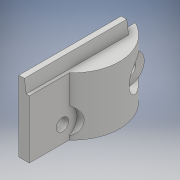
# Autodesk Inventor part: Faceplatev11
Saved by Autodesk Inventor 2017 (Build 210142000, 142)
## iProperties
Created: 2017-12-13
Part Number: Faceplatev11
Material: Generic
Document SubType Name: Modeling
Designer: andrew
Density: 1 g/cm^3
Appearance: Default
Author: andrew
Autodesk Inventor part; units mm, degrees
ref_plane "YZ Plane" through (0, 0, 0) normal (1, 0, 0) x (0, 1, 0)
ref_plane "XZ Plane" through (0, 0, 0) normal (0, 1, 0) x (-1, 0, 0)
ref_plane "XY Plane" through (0, 0, 0) normal (0, 0, 1) x (1, 0, 0)
sketch "Sketch1" plane through (0, 0, 0) normal (0, 0, 1) x (1, 0, 0)
  arc A0 (2, -4.031129) -> (2, 4.031129) centre (0, 0) ccw
  line L0 (2, -4.031129) -> (2, -1.999397)
  line L1 (2, 2.000654) -> (2, 4.031129)
  line L2 (2, 2.000654) -> (2, -1.999397)
  constraints: 6 end point, 2 point on circle, 1 centre point, 1 vertical
extrude "Extrusion1" add sketch "Sketch1" along normal blind 7.3
sketch "Sketch2" plane through (0, 0, 7.3) normal (0, 0, 1) x (1, 0, 0)
  arc A0 (2, -4.031129) -> (2, 4.031129) centre (0, 0) ccw
  line L0 (2, 4.031129) -> (2, 2.681129)
  line L1 (2, 4.031129) -> (2, -4.031129)
  line L2 (2, 2.681129) -> (3.614076, 2.681129)
  dimension "d2" = 1.35
  constraints: 4 end point, 1 horizontal, 1 point on circle, 1 point on line
  measures "d2" distance of L0.start L0.end
extrude "Extrusion2" cut sketch "Sketch2" against normal blind 1.5 contours L2 L0 A0
sketch "Sketch3" plane through (2, -4.031129, 0) normal (-1, 0, 0) x (0, 0, 1)
  line L0 (0, 8.062258) -> (5.8, 8.062258)
  arc A0 (3.793007, 1.425366) -> (3.791184, 0.225367) centre (3.792095, 0.825367) ccw
  line L1 (6.969827, -1.268871) -> (2.357408, -1.268871)
  line L2 (3.791184, 0.225367) -> (6.492703, 0.221263)
  line L3 (6.494526, 1.421261) -> (3.793007, 1.425366)
  arc A1 (6.492703, 0.221263) -> (7.291127, 0.185183) centre (6.892703, 0.220655) ccw
  line L4 (7.291127, 0.185183) -> (7.291127, 1.472687)
  line L5 (7.3, 4.997606) -> (7.3, 6.564652)
  line L6 (2.357408, -1.268871) -> (2.357408, -1.968871)
  circle A2 centre (1.793923, 0.031129) radius 0.6
  line L7 (0, 2.030475) -> (0, 0)
  line L8 (0, -1.968871) -> (2.357408, -1.968871)
  line L9 (0, 0) -> (0, -1.968871)
  arc A3 (7.291127, 1.472687) -> (6.494526, 1.421261) centre (6.894526, 1.420654) ccw
  line L10 (7.3, 0) -> (7.3, 4.997606)
  arc A4 (6.793923, 5.531129) -> (5.945395, 6.379657) centre (6.369659, 5.955393) ccw
  line L11 (2.551282, 1.288488) -> (6.793923, 5.531129)
  arc A5 (0.793315, 1.629923) -> (1.193922, 2.029315) centre (0.793923, 2.029923) ccw
  line L12 (0.393316, 1.630531) -> (0.793315, 1.629923)
  arc A6 (0, 2.030475) -> (0.393316, 1.630531) centre (0.4, 2.030475) ccw
  circle A7 centre (3.18453, 6.515928) radius 0.6
  line L13 (5.945395, 6.379657) -> (1.702754, 2.137016)
  line L14 (1.193922, 2.029315) -> (1.2, 6.029311)
  arc A8 (1.2, 6.029311) -> (0.800608, 6.429918) centre (0.8, 6.029918) ccw
  line L15 (0.800608, 6.429918) -> (0.400609, 6.430525)
  arc A9 (0.400609, 6.430525) -> (0, 6.030526) centre (0.4, 6.030526) ccw
  line L16 (0, 8.062258) -> (0, 6.030526)
  arc A10 (1.702754, 2.137016) -> (2.551282, 1.288488) centre (2.127018, 1.712752) ccw
  line L17 (5.8, 8.062258) -> (5.8, 7.213109)
  line L18 (5.8, 7.213109) -> (7.3, 7.213109)
  line L19 (7.3, 6.564652) -> (7.3, 7.213109)
  line L20 (8.3, 0) -> (7.3, 0)
  line L21 (8.3, -1.968871) -> (8.3, 0)
  line L22 (6.969827, -1.968871) -> (8.3, -1.968871)
  line L23 (6.969827, -1.968871) -> (6.969827, -1.268871)
  line L24 (0, 8.062258) -> (0, 0)
  line L25 (0, 0) -> (0, 8.062258)
  line L26 (0, 8.062258) -> (0, 4.031129)
  line L27 (0, 4.031129) -> (-3.475926, 4.031129)
  circle A11 centre (3.18453, 6.515928) radius 1.416868
  circle A12 centre (1.793923, 0.031129) radius 1.416868
  point P0 (7.3, 0.966477)
  point P1 (0, 4.031129)
  point P2 (5.8, 6.712258)
  dimension "d11" = 2.83374
  dimension "d7" = 1.2
  dimension "d8" = 1.2
  dimension "d10" = 2.83374
  constraints: 54 end point, 18 point on circle, 12 centre point, 1 coincident, 1 horizontal, 1 midpoint, 1 vertical, 3 other
  measures "d7" diameter of A2
  measures "d8" diameter of A7
  measures "d10" diameter of A11
extrude "Extrusion3" add sketch "Sketch3" against normal blind 2.38 contours A12 A10 | A12 A10 | A11
sketch "Sketch4" plane through (4.38, 2.484799, 3.18453) normal (1, 0, 0) x (0, 0, -1)
  spline S0 degree 5 poles (-0.6, 0) (-0.6, 0.115203) (-0.572174, 0.228108) (-0.519386, 0.330757) (-0.445495, 0.417191) (-0.294999, 0.527814) (-0.227367, 0.5631) (-0.154009, 0.587492) (-0.077351, 0.599909) (0.120646, 0.600142) (0.242119, 0.569441) (0.350015, 0.508794) (0.438267, 0.426407) (0.53365, 0.280074) (0.559074, 0.228631) (0.578437, 0.174164) (0.591252, 0.117527) (0.607151, -0.0418) (0.595965, -0.147298) (0.561126, -0.249394) (0.504475, -0.341173) (0.36418, -0.486765) (0.282308, -0.542829) (0.191193, -0.581079) (0.095541, -0.6) (-0.185719, -0.6) (-0.370669, -0.529641) (-0.527767, -0.380653) (-0.6, -0.186699) (-0.6, 0) knots 0 0 0 0 0 0 0.15157455 0.15157455 0.15157455 0.15157455 0.25307731 0.25307731 0.25307731 0.25307731 0.41378439 0.41378439 0.41378439 0.41378439 0.49116677 0.49116677 0.49116677 0.49116677 0.62653879 0.62653879 0.62653879 0.62653879 0.75339947 0.75339947 0.75339947 0.75339947 1 1 1 1 1 1
  circle A0 centre (1.390607, -6.484799) radius 0.6
  point P0 (3.18453, -2.484799)
  constraints: 1 other
extrude "Extrusion4" cut sketch "Sketch4" against normal blind 5
sketch "Sketch5" plane through (0, 0, 7.3) normal (0, 0, 1) x (1, 0, 0)
  line L0 (3.614076, 2.681129) -> (2, 2.681129)
  line L1 (2, 2.681129) -> (3.182, 2.681129)
  line L2 (3.182, -3.928209) -> (2, -3.928209)
  line L3 (2, -3.928209) -> (2, 2.681129)
  line L4 (3.182, -3.928209) -> (5.945159, -3.928209)
  line L5 (5.945159, -3.928209) -> (5.945159, 3.167221)
  line L6 (5.945159, 3.167221) -> (3.193824, 3.167221)
  line L7 (3.193824, 3.167221) -> (2.705649, 3.167221)
  line L8 (3.193824, 3.167221) -> (3.682, 3.167221) construction
  line L9 (2.705649, -3.928209) -> (2.705649, 3.167221)
  line L10 (2.705649, -3.928209) -> (9.801079, -3.928209) construction
  point P0 (0, 0)
  dimension "d15" = 1.182
  dimension "d23" = 180
  dimension "d44" = 90
  constraints: 20 end point, 5 horizontal, 2 equal length, 2 parallel, 2 point on line, 1 perpendicular
  measures "d15" distance of L2.start L2.end
  measures "d23" angle of L7 L8
  measures "d44" angle of L10 L9
extrude "Extrusion5" cut sketch "Sketch5" against normal blind 1.5 contours L9 L7 L6 L5 L4 L2
sketch "Sketch6" plane through (2, -4.031129, 0) normal (-1, 0, 0) x (0, 0, 1)
  line L0 (7.3, 0) -> (7.225, 0)
  line L1 (7.225, 0) -> (7.225, 6.712258)
  line L2 (7.225, 6.712258) -> (7.3, 6.712258)
  line L3 (7.3, 6.712258) -> (7.3, 0)
  line L4 (0, 8.062258) -> (0.075, 8.062258)
  line L5 (0.075, 8.062258) -> (0.075, -1.050881)
  line L6 (0.075, -1.050881) -> (0, -1.050881)
  line L7 (0, -1.050881) -> (0, 8.062258)
  point P0 (0, 4.031129)
  dimension "d18" = 0.075
  dimension "d19" = 0.075
  constraints: 16 end point, 4 parallel, 2 horizontal, 2 perpendicular
  measures "d18" distance of L1.end L2.end
  measures "d19" distance of L5.end L6.end
extrude "Extrusion6" cut sketch "Sketch6" against normal blind 10
sketch "Sketch7" plane through (4.38, -4, 1.793923) normal (1, 0, 0) x (0, 0, -1)
  circle A0 centre (0, 0) radius 0.6
  circle A1 centre (0, 0) radius 1.416868
  circle A2 centre (-1.390607, 6.484799) radius 0.6
  circle A3 centre (-1.390607, 6.484799) radius 1.416868
  point P0 (1.793923, 4)
extrude "Extrusion7" cut sketch "Sketch7" against normal blind 1.38
sketch "Sketch8" plane through (2, 2.681129, 5.8) normal (-1, 0, 0) x (0, 0, 1)
  line L0 (-5.800031, 1.35) -> (-0.000031, 1.35) construction
  line L1 (-5.800031, 1.35) -> (-5.800031, -0.681732) construction
  arc A0 (1.491127, -5.239571) -> (0.694526, -5.290997) centre (1.094526, -5.291604) ccw construction
  line L2 (1.491127, -6.527075) -> (1.491127, -5.239571) construction
  line L3 (1.499969, -6.712258) -> (1.499969, -1.714651) construction
  arc A1 (0.993923, -1.181129) -> (0.145395, -0.332601) centre (0.569659, -0.756865) ccw construction
  line L4 (-0.000031, 1.35) -> (-0.000031, 0.500852) construction
  line L5 (1.499969, -0.147606) -> (1.499969, 0.500852) construction
  arc A2 (-5.399423, -0.281733) -> (-5.800031, -0.681732) centre (-5.400031, -0.681732) ccw construction
  line L6 (-4.999423, -0.28234) -> (-5.399423, -0.281733) construction
  arc A3 (-4.600031, -0.682947) -> (-4.999423, -0.28234) centre (-5.000031, -0.68234) ccw construction
  circle A4 centre (-2.61547, -0.19633) radius 0.6 construction
  line L7 (-4.606109, -4.682943) -> (-4.600031, -0.682947) construction
  line L8 (1.499969, -1.714651) -> (1.499969, -0.147606) construction
  arc A5 (-2.006993, -5.286892) -> (-2.008816, -6.486891) centre (-2.007905, -5.886891) ccw construction
  line L9 (0.694526, -5.290997) -> (-2.006993, -5.286892) construction
  line L10 (-3.248718, -5.42377) -> (0.993923, -1.181129) construction
  line L11 (-2.008816, -6.486891) -> (0.692703, -6.490995) construction
  line L12 (1.169796, -7.981129) -> (-3.442623, -7.981129) construction
  line L13 (0.145395, -0.332601) -> (-4.097246, -4.575242) construction
  line L14 (-3.442623, -7.981129) -> (-3.442623, -8.681129) construction
  circle A6 centre (-4.006077, -6.681129) radius 0.6
  line L15 (-5.800031, -4.681783) -> (-5.800031, -6.712258) construction
  line L16 (-5.800031, -8.681129) -> (-3.442623, -8.681129) construction
  line L17 (-5.800031, -6.712258) -> (-5.800031, -8.681129) construction
  arc A7 (-5.800031, -4.681783) -> (-5.406715, -5.081727) centre (-5.400031, -4.681783) ccw construction
  arc A8 (-5.006716, -5.082335) -> (-4.606109, -4.682943) centre (-5.006108, -4.682335) ccw construction
  arc A9 (-4.097246, -4.575242) -> (-3.248718, -5.42377) centre (-3.672982, -4.999506) ccw construction
  line L18 (-5.406715, -5.081727) -> (-5.006716, -5.082335) construction
  line L19 (-0.000031, 0.500852) -> (1.499969, 0.500852) construction
  arc A10 (0.692703, -6.490995) -> (1.491127, -6.527075) centre (1.092703, -6.491603) ccw construction
  line L20 (2.499969, -6.712258) -> (1.499969, -6.712258) construction
  line L21 (1.169796, -8.681129) -> (1.169796, -7.981129) construction
  line L22 (2.499969, -8.681129) -> (2.499969, -6.712258) construction
  line L23 (1.169796, -8.681129) -> (2.499969, -8.681129) construction
  line L24 (-5.8, 1.35) -> (-5.8, 6.712258) construction
  line L25 (-5.8, 6.712258) -> (-5.8, 1.35) construction
  line L26 (-5.8, 1.35) -> (-5.8, 4.031129) construction
  line L27 (-5.8, 4.031129) -> (-9.275926, 4.031129) construction
  circle A11 centre (-2.61547, -0.19633) radius 1.416868 construction
  circle A12 centre (-4.006108, -6.681129) radius 1.416868 construction
  circle A13 centre (-4.006077, -6.681129) radius 0.6 construction
  line L28 (-5.725, 1.35) -> (-5.725, -6.712258) construction
  line L29 (1.425, -6.712258) -> (1.425, 0) construction
  line L30 (-5.725031, -8.681129) -> (1.425, -8.681129)
  line L31 (1.425, -8.681129) -> (1.425, -5.292106)
  line L32 (1.425, -5.292106) -> (-5.725031, -5.292106)
  line L33 (-5.725031, -5.292106) -> (-5.725031, -8.681129)
  point P0 (-5.8, -2.681129)
  point P1 (1.5, -5.74578)
  point P2 (-5.8, -2.681129)
  point P3 (0, 0)
  dimension "d29" = 2.83374
  dimension "d26" = 1.2
  dimension "d27" = 1.2
  dimension "d28" = 2.83374
  constraints: 64 end point, 18 point on circle, 12 centre point, 2 horizontal, 2 parallel, 2 point on line, 1 coincident, 1 midpoint, 1 perpendicular, 1 vertical, 3 other
  measures "d26" diameter of A6
  measures "d27" diameter of A4
  measures "d28" diameter of A11
extrude "Extrusion8" add sketch "Sketch8" against normal blind 1
sketch "Sketch11" plane through (2, -6, 0.074969) normal (0, -1, 0) x (1, 0, 0)
  line L0 (0.705649, 5.725031) -> (1, 5.725031) construction
  line L1 (0.705649, 7.150031) -> (0.705649, 5.725031) construction
  line L2 (0.705649, 7.150031) -> (1, 7.150031) construction
  line L3 (1, 5.725031) -> (1, 7.150031) construction
  line L4 (0.705649, 7.150031) -> (0.705649, 5.725031)
  line L5 (0.705649, 7.150031) -> (0.505649, 7.150031)
  line L6 (0, 7.150031) -> (0.705649, 7.150031)
  line L7 (0.705649, 7.150031) -> (0.905649, 7.150031) construction
  line L8 (0.505649, 7.150031) -> (0.705649, 5.725031)
  line L9 (0.705649, 5.725031) -> (1, 5.725031)
  line L10 (0.705649, 5.725031) -> (1, 5.725031)
  line L11 (1, 5.725031) -> (1, 7.150031)
  line L12 (1, 5.725031) -> (1, 7.150031)
  line L13 (1, 7.150031) -> (0.505649, 7.150031)
  point P0 (-2, -0.074969)
  dimension "d45" = 0.2
  dimension "d46" = 180
  constraints: 12 end point, 4 collinear, 1 horizontal, 1 perpendicular
  measures "d45" distance of L1.start L5.end
  measures "d46" angle of L5 L7
extrude "Extrusion10" cut sketch "Sketch11" against normal blind 10
sketch "Sketch12" plane through (2, 2.681129, 5.8) normal (-1, 0, 0) x (0, 0, 1)
  line L0 (-5.8, 1.35) -> (0, 1.35)
  line L1 (1.491127, -6.527075) -> (1.491127, -5.239571)
  line L2 (1.5, -6.712258) -> (1.5, -1.714651)
  arc A0 (0.993923, -1.181129) -> (0.145395, -0.332601) centre (0.569659, -0.756865) ccw
  line L3 (0, 1.35) -> (0, 0.500852)
  line L4 (1.5, -0.147606) -> (1.5, 0.500852)
  arc A1 (-5.399391, -0.281733) -> (-5.8, -0.681732) centre (-5.4, -0.681732) ccw
  line L5 (-4.999392, -0.28234) -> (-5.399391, -0.281733)
  arc A2 (-4.6, -0.682947) -> (-4.999392, -0.28234) centre (-5, -0.68234) ccw
  circle A3 centre (-2.61547, -0.19633) radius 0.6
  line L6 (-4.606078, -4.682943) -> (-4.6, -0.682947)
  line L7 (1.5, -1.714651) -> (1.5, -0.147606)
  arc A4 (-2.006993, -5.286892) -> (-2.008816, -6.486891) centre (-2.007905, -5.886891) ccw
  line L8 (1.491127, -5.292207) -> (-2.006993, -5.286892)
  line L9 (-3.248718, -5.42377) -> (0.993923, -1.181129)
  line L10 (-2.008816, -6.486891) -> (1.491127, -6.492208)
  line L11 (1.169827, -7.981129) -> (-3.442592, -7.981129)
  line L12 (0.145395, -0.332601) -> (-4.097246, -4.575242)
  line L13 (-3.442592, -7.981129) -> (-3.442592, -8.681129)
  circle A5 centre (-4.006077, -6.681129) radius 0.6
  line L14 (-5.8, -8.681129) -> (-3.442592, -8.681129)
  line L15 (-5.8, -6.712258) -> (-5.8, -8.681129)
  arc A6 (-5.8, -4.681783) -> (-5.406684, -5.081727) centre (-5.4, -4.681783) ccw
  arc A7 (-5.006685, -5.082335) -> (-4.606078, -4.682943) centre (-5.006077, -4.682335) ccw
  arc A8 (-4.097246, -4.575242) -> (-3.248718, -5.42377) centre (-3.672982, -4.999506) ccw
  line L16 (-5.406684, -5.081727) -> (-5.006685, -5.082335)
  line L17 (0, 0.500852) -> (1.5, 0.500852)
  line L18 (2.5, -6.712258) -> (1.5, -6.712258)
  line L19 (1.169827, -8.681129) -> (1.169827, -7.981129)
  line L20 (2.5, -8.681129) -> (2.5, -6.712258)
  line L21 (1.169827, -8.681129) -> (2.5, -8.681129)
  circle A9 centre (-2.61547, -0.19633) radius 1.416868
  circle A10 centre (-4.006077, -6.681129) radius 1.416868
  circle A11 centre (-4.006077, -6.681129) radius 0.6
  line L22 (-5.8, -4.681783) -> (-5.8, -0.681732)
  point P0 (1.5, -5.74578)
  point P1 (0, 0)
  dimension "d52" = 2.83374
  dimension "d49" = 1.2
  dimension "d50" = 1.2
  dimension "d51" = 2.83374
  constraints: 46 end point, 14 point on circle, 10 centre point, 2 point on line, 1 coincident, 1 tangent, 1 vertical, 3 other
  measures "d49" diameter of A5
  measures "d50" diameter of A3
  measures "d51" diameter of A9
extrude "Extrusion11" [suppressed]
sketch "Sketch13" plane through (2, 2.681129, 5.8) normal (-1, 0, 0) x (0, 0, 1)
  circle A0 centre (-4.006077, -6.681129) radius 0.6 construction
  line L0 (1.425, -8.681129) -> (1.425, 0)
  line L1 (1.425, 0) -> (0, 0) construction
  line L2 (0, 0) -> (0, 1.35) construction
  line L3 (-5.725, 1.35) -> (0, 1.35) construction
  line L4 (-5.725, 1.35) -> (-5.725, -5.292106)
  line L5 (-5.725, -5.292106) -> (-5.725031, -5.292106)
  line L6 (-5.725031, -5.292106) -> (-5.725031, -8.681129)
  line L7 (-5.725031, -8.681129) -> (1.425, -8.681129) construction
  line L8 (1.425, 0) -> (1.325, 0)
  line L9 (1.325, 0) -> (1.325, -8.954641)
  line L10 (1.325, -8.954641) -> (1.425, -8.954641)
  line L11 (1.425, -8.954641) -> (1.425, 0)
  line L12 (-5.725, 1.35) -> (-5.625, 1.35)
  line L13 (-5.625, 1.35) -> (-5.625, -8.82591)
  line L14 (-5.625, -8.82591) -> (-5.725, -8.82591)
  line L15 (-5.725, -8.82591) -> (-5.908892, -8.82591)
  line L16 (-5.908892, -8.82591) -> (-5.908892, 1.35)
  line L17 (-5.908892, 1.35) -> (-5.725, 1.35)
  point P0 (-5.8, -2.681129)
  dimension "d55" = 0.1
  dimension "d56" = 0.1
  constraints: 20 end point, 4 perpendicular, 3 horizontal, 3 parallel, 1 other
  measures "d55" distance of L10.end L9.end
  measures "d56" distance of L13.end L14.end
extrude "Extrusion12" cut sketch "Sketch13" against normal blind 10
sketch "Sketch14" plane through (2.705649, -6, 5.8) normal (0, -1, 0) x (1, 0, 0)
  line L0 (-0.185965, 1.325) -> (-0.705649, 1.325)
  line L1 (-0.705649, -5.625) -> (-0.705649, 1.325)
  line L2 (-0.705649, -5.625) -> (0.294351, -5.625)
  line L3 (0.294351, 0) -> (0.294351, -5.625)
  line L4 (0.294351, 0) -> (0, 0)
  line L5 (0, 0) -> (-0.185965, 1.325)
extrude "Extrusion13" add sketch "Sketch14" along normal blind 1.2
sketch "Sketch15" plane through (2, 2.681129, 5.8) normal (-1, 0, 0) x (0, 0, 1)
  line L0 (1.325, 0) -> (1.325, -9.881129)
  line L1 (1.325, 0) -> (1.225, 0)
  line L2 (1.225, 0) -> (1.225, -10.734444)
  line L3 (1.225, -10.734444) -> (1.325, -10.734444)
  line L4 (1.325, -10.734444) -> (1.325, 0)
  point P0 (-5.8, -2.681129)
  dimension "d61" = 0.1
  constraints: 8 end point, 2 parallel, 1 horizontal, 1 perpendicular
  measures "d61" distance of L3.end L2.end
extrude "Extrusion14" cut sketch "Sketch15" against normal blind 10
equation "\"d10\" = d11"
equation "\"d28\" = d29"
equation "\"d51\" = d52"
body "Solid1" dims "d61" = 0.1
